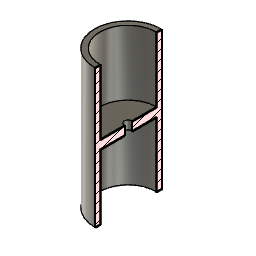
coupler (4.3mm gap) v5 (Autodesk Fusion 360 design; units mm, degrees)
Autodesk Fusion 360 part; units mm, degrees
sketch "Sketch1" plane through (0, 0, 0) normal (0, 0, 1) x (1, 0, 0)
  circle A0 centre (0, 0) radius 19.305
  circle A1 centre (0, 0) radius 16.25
  dimension "d1" = 38.61
  dimension "d9" = 32.5
  constraint coincident A0.centre A1.centre
  measures "d1" diameter of A0
  measures "d9" diameter of A1
extrude "Extrude1" add sketch "Sketch1" along normal blind 80 makes body 1
ref_plane "WorkPlane1" through (0, 0, 40) normal (0, 0, 1) x (1, 0, 0)
sketch "Sketch2" plane through (0, 0, 40) normal (0, 0, 1) x (1, 0, 0)
  circle A0 centre (0, 0) radius 18.6687
  circle A1 centre (0, 0) radius 2.15
  dimension "d6" = 4.3
  constraint coincident A0.centre A1.centre
  constraint concentric A0 A1
  measures "d6" diameter of A1
extrude "Extrude2" add sketch "Sketch2" along normal mid plane 5 separate body makes body 2
combine "Combine1" operation add target body 1 tool bodies 2
